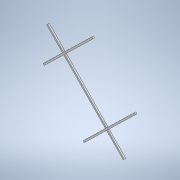
# Autodesk Inventor part: print009_Guss_innen_erweitert
Saved by Autodesk Inventor 2020.3 (Build 243373000, 373)
## iProperties
Created: 2020-03-04
Part Number: print009_Guss_innen_erweitert
Material: Generic
Document SubType Name: Modeling
Designer: Mara
Density: 1 g/cm^3
Appearance: Default
Mass: 1.1982 g
Surface Area: 24.0527 cm^2
Volume: 1.1982 cm^3
Author: Mara
Autodesk Inventor part; units mm, degrees
ref_plane "YZ Plane" through (0, 0, 0) normal (1, 0, 0) x (0, 1, 0)
ref_plane "XZ Plane" through (0, 0, 0) normal (0, 1, 0) x (-1, 0, 0)
ref_plane "XY Plane" through (0, 0, 0) normal (0, 0, 1) x (1, 0, 0)
sketch "Sketch1" plane through (0, 0, 0) normal (0, 0, 1) x (1, 0, 0)
  arc A0 (5.5811, -56.8606) -> (20.209, -64.6836) centre (38.8796, -12.1848) ccw construction
  arc A1 (-7.6539, -43.4667) -> (5.5811, -56.8606) centre (37.8873, -11.7018) ccw construction
  arc A2 (-7.6539, -43.4667) -> (-31.2183, -12.0793) centre (-386.265, -303.1724) ccw construction
  arc A3 (-31.2183, -12.0793) -> (-63.3277, 19.0744) centre (-191.6112, -145.2692) ccw construction
  arc A4 (-67.5206, 26.3221) -> (-63.3277, 19.0744) centre (-54.6162, 28.9507) ccw construction
  arc A5 (-66.9469, 41.0059) -> (-67.5206, 26.3221) centre (-15.6776, 31.6496) ccw construction
  line L0 (-66.9469, 41.0059) -> (-50.7446, 56.9005) construction
  arc A6 (-3.6955, 79.7027) -> (-26.0985, 81.0785) centre (-17.6076, 36.2535) ccw construction
  arc A7 (1.4491, 74.6716) -> (-3.6955, 79.7027) centre (-6.1453, 72.0517) ccw construction
  arc A8 (2.6831, 69.1533) -> (1.4491, 74.6716) centre (-18.5892, 67.2935) ccw construction
  arc A9 (2.6831, 69.1533) -> (3.1898, 63.5624) centre (229.5421, 86.8959) ccw construction
  arc A10 (3.1898, 63.5624) -> (8.7161, 49.818) centre (30.4167, 66.5265) ccw construction
  arc A11 (8.7161, 49.818) -> (19.0471, 39.3259) centre (47.1297, 77.3097) ccw construction
  arc A12 (19.0471, 39.3259) -> (32.6891, 29.8296) centre (104.4845, 147.5139) ccw construction
  arc A13 (32.6891, 29.8296) -> (50.5655, 19.6706) centre (502.3948, 835.5524) ccw construction
  arc A14 (57.8671, 12.5741) -> (50.5655, 19.6706) centre (33.0101, -5.6965) ccw construction
  arc A15 (67.0572, -4.125) -> (57.8671, 12.5741) centre (18.4686, -19.9867) ccw construction
  arc A16 (68.9532, -23.0115) -> (67.0572, -4.125) centre (24.8632, -17.8992) ccw construction
  line L1 (-52.1723, 55.4999) -> (-51.76, 55.076) construction
  line L2 (43.4701, -39.9764) -> (43.0518, -39.5463) construction
  line L3 (42.0363, -41.3708) -> (43.4701, -39.9764) construction
  line L4 (-4.1456, -47.7345) -> (58.0182, 12.7211)
  line L5 (56.6239, 14.1548) -> (-5.54, -46.3007)
  line L6 (-55.3767, 12.3052) -> (3.7843, 69.8404)
  line L7 (2.3899, 71.2742) -> (-56.7711, 13.739)
  line L8 (-56.7711, 13.739) -> (-55.3767, 12.3052)
  line L9 (2.3899, 71.2742) -> (3.7843, 69.8404)
  line L10 (-52.1723, 55.4999) -> (-50.7446, 56.9005) construction
  line L11 (-4.1456, -47.7345) -> (-5.54, -46.3007)
  line L12 (58.0182, 12.7211) -> (56.6239, 14.1548)
  line L13 (-51.76, 55.076) -> (-50.3262, 56.4704)
  line L14 (41.618, -40.9406) -> (43.0518, -39.5463)
  line L15 (-51.76, 55.076) -> (41.618, -40.9406)
  line L16 (-50.3262, 56.4704) -> (-50.7446, 56.9005) construction
  line L17 (-50.7446, 56.9005) -> (-26.0985, 81.0785) construction
  line L18 (43.0518, -39.5463) -> (-50.3262, 56.4704)
  line L19 (41.618, -40.9406) -> (42.0363, -41.3708) construction
  point P0 (0, 0)
  point P1 (-8.2693, 4.2237)
  point P2 (-4.9861, 4.7501)
  point P3 (-66.0155, 22.3561)
  point P4 (24.203, -20.1649)
  point P5 (22.8086, -18.7311)
  point P6 (-30.7071, 36.2969)
  point P7 (-32.1015, 37.7306)
  point P8 (-33.5353, 36.3363)
  point P9 (-32.1409, 34.9025)
  point P10 (21.3749, -20.1255)
  point P11 (22.7692, -21.5593)
  point P12 (22.8086, -18.7311)
  point P13 (-30.7071, 36.2969)
  point P14 (-32.1409, 34.9025)
  point P15 (21.3749, -20.1255)
  point P16 (24.203, -20.1649)
  point P17 (22.7692, -21.5593)
  point P18 (-33.5353, 36.3363)
  point P19 (-32.1015, 37.7306)
  dimension "d244" = 2
  dimension "d245" = 2
  dimension "d251" = 0.6
  dimension "d252" = 0.6
  dimension "d253" = 2
  constraints: 40 end point, 36 point on circle, 24 parallel, 17 centre point, 12 perpendicular, 2 collinear, 2 point on line, 2 tangent, 24 other
  measures "d244" distance between parallel lines of L5 L4
  measures "d245" distance between parallel lines of L7 L6
  measures "d251" distance between parallel lines of L3 L14
  measures "d252" distance of L0.end L13.end
  measures "d253" distance between parallel lines of L18 L15
extrude "Extrusion12" add sketch "Sketch1" along normal blind 2
move faces "Move1" translate (1.7922, 1.743, 0) faces at (3.3195, 70.3184, 0.6667)
move faces "Move2" translate (1.7922, 1.743, 0) faces at (57.5534, 13.199, 0.6667)
move faces "Move3" translate (-1.7922, -1.743, 0) faces at (-4.6104, -47.2565, 1.3333)
move faces "Move4" translate (-1.7922, -1.743, 0) faces at (-56.3063, 13.2611, 0.6667)
move faces "Move5" translate (-2.1613, 2.2224, 0) faces at (-50.8042, 56.0056, 0.6667)
move faces "Move6" translate (2.4402, -2.5091, 0) faces at (42.0959, -40.4758, 0.6667)
body "Solid4"
